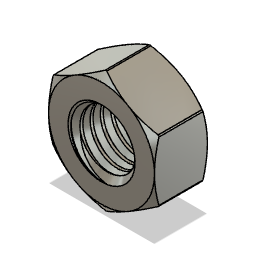
M8 Nut v5 (Autodesk Fusion 360 design; units mm, degrees)
Autodesk Fusion 360 part; units mm, degrees
sketch "Skizze1" plane through (0, 0, 0) normal (0, 0, 1) x (1, 0, 0)
  line L0 (-6.5, -3.7528) -> (0, -7.5056)
  line L1 (0, -7.5056) -> (6.5, -3.7528)
  line L2 (6.5, -3.7528) -> (6.5, 3.7528)
  line L3 (6.5, 3.7528) -> (0, 7.5056)
  line L4 (0, 7.5056) -> (-6.5, 3.7528)
  line L5 (-6.5, 3.7528) -> (-6.5, -3.7528)
  dimension "d3" = 6.5
  constraint vertical L5
  measures "d3" distance of origin L5
extrude "Extrusion1" add sketch "Skizze1" along normal mid plane 6.5
sketch "Skizze2" plane through (0, 0, 3.25) normal (0, 0, 1) x (1, 0, 0)
  line L0 (-6.5, 3.7528) -> (-6.5, -3.7528)
  line L1 (-6.5, -3.7528) -> (0, -7.5056)
  line L2 (0, -7.5056) -> (6.5, -3.7528)
  line L3 (6.5, -3.7528) -> (6.5, 3.7528)
  line L4 (6.5, 3.7528) -> (0, 7.5056)
  line L5 (0, 7.5056) -> (-6.5, 3.7528)
hole "Bohrung1" at (0, 0, 3.25) direction (0, 0, -1) diameter 6.78 end through all
thread "Gewinde1" "ISO Metric profile 8.0 M8x1.25 6H" major diameter 8.17 minor diameter 6.7795 pitch 1.25 angle 60 modelled right hand crest width 0.343 on face at (0.3375, -3.3732, -1.0833) crest through (3.3898, 0, 2.9375)
sketch "Skizze4" plane through (0, 0, 0) normal (1, 0, 0) x (0, 0, -1)
  line L0 (3.25, 3.7528) -> (3.25, 7.5056)
  line L1 (3.25, -3.7528) -> (3.25, 3.7528) construction
  line L2 (3.25, -7.5056) -> (3.25, -3.7528)
  line L3 (3.25, 7.5056) -> (-3.25, 7.5056)
  line L4 (2.6726, 7.5056) -> (3.25, 6.5056)
  line L5 (3.25, 7.5056) -> (2.817, 7.2556) construction
  line L6 (3.25, 6.5056) -> (3.25, 0)
  line L7 (2.6726, 7.5056) -> (0, 7.5056)
  line L8 (0, 1.75) -> (0, 22.5) construction
  line L9 (-2.6726, 7.5056) -> (0, 7.5056)
  line L10 (-2.6726, 7.5056) -> (-3.25, 6.5056)
  line L11 (-3.25, 6.5056) -> (-3.25, 0)
  line L12 (-3.25, 0) -> (3.25, 0)
  line L13 (-3.25, 8.5056) -> (0, 8.5056)
  line L14 (3.25, 8.5056) -> (0, 8.5056)
  line L15 (3.25, 8.5056) -> (4.25, 6.7735)
  line L16 (4.25, 6.7735) -> (4.25, -1)
  line L17 (-4.25, -1) -> (4.25, -1)
  line L18 (-4.25, 6.7735) -> (-4.25, -1)
  line L19 (-3.25, 8.5056) -> (-4.25, 6.7735)
  line L20 (-3.25, 0) -> (-4.25, 0)
  line L21 (3.25, 0) -> (4.25, 0)
  dimension "d18" = 0.5
  dimension "d19" = 1
  dimension "d23" = 150
  constraint coincident L3 L4.start
  constraint coincident L0 L4.end
  constraint coincident L0.end L3.start
  constraint midpoint L1 L6.end
  constraint midpoint L3 L7.end
  constraint symmetric L4.start L8 L9.start
  constraint symmetric L4.end L8 L10.end
  constraint symmetric L6.end L8 L11.end
  constraint symmetric L7.end L8 L9.end
  constraint coincident L18 L20.end
  constraint perpendicular L18 L20
  constraint coincident L16 L21.end
  constraint perpendicular L16 L21
  constraint perpendicular L4 L5
  constraint coincident L4 L5.end
  measures "d18" distance of L0.end L5.end
  measures "d23" angle of L4 L6
revolve "Drehen1" cut sketch "Skizze4" angle 360 about axis through (0, 0, 1.75) along (0, 0, 1) contours L0 L3 L6 L7 L9 L10 L11 L13 L14 L15 L16 L18 L19 L20 L21 | L0 L3 L4
fillet "Abrundung1" radius 0.2 6 edges at (6.5, 3.7528, 0) (6.5, -3.7528, 0) (0, -7.5056, 0) (-6.5, -3.7528, 0) (0, 7.5056, 0) (-6.5, 3.7528, 0)
sketch "Skizze5" plane through (0, 0, 0) normal (1, 0, 0) x (0, 0, -1)
  line L0 (-3.25, 4.1071) -> (-2.5429, 3.4)
  line L1 (-2.5429, 3.4) -> (0, 3.4)
  line L2 (0, 1.75) -> (0, 22.5)
  line L3 (0, 3.4) -> (0, 0) construction
  line L4 (-2.5429, 3.4) -> (-3.25, 3.4) construction
  line L5 (-3.25, 3.4) -> (-2.8964, 3.7536) construction
  line L6 (-3.25, 4.1071) -> (-3.25, 0)
  line L7 (-3.25, 0) -> (0, 0)
  line L8 (2.5429, 3.4) -> (0, 3.4)
  line L9 (3.25, 4.1071) -> (2.5429, 3.4)
  line L10 (3.25, 4.1071) -> (3.25, 0)
  line L11 (3.25, 0) -> (0, 0)
  line L12 (-3.25, -5.7635) -> (-3.25, -6.5056)
  line L13 (-3.25, -0.2687) -> (-3.25, -5.4948)
  line L14 (-3.25, 5.4948) -> (-3.25, 0.2687)
  line L15 (-3.25, 6.5056) -> (-3.25, 5.7635)
  line L16 (-3.25, 5.4948) -> (-3.25, 0.2687)
  line L17 (-3.25, -0.2687) -> (-3.25, -5.4948)
  dimension "d28" = 3.4
  dimension "d29" = 0.5
  dimension "d31" = 45
  constraint horizontal L1
  constraint coincident L1.end L2
  constraint coincident L3.end L7.end
  constraint coincident L0 L5.end
  constraint perpendicular L0 L5
  constraint symmetric L0.start L2 L9.start
  constraint symmetric L0.end L2 L8.start
  constraint symmetric L1.end L2 L3.start
  constraint symmetric L2 L6.end L10.end
  constraint symmetric L2 L3.end L7.end
  constraint horizontal L7
  constraint vertical L6
  constraint horizontal L4
  constraint coincident L4.end L6
  constraint collinear L6 L14
  measures "d28" distance of L1.end L3.end
  measures "d29" distance of L4.end L5.end
  measures "d31" angle of L0 L6
revolve "Drehen2" cut sketch "Skizze5" angle 360 about axis through (0, 0, 1.75) along (0, 0, 1)
equation "HexWidth = 13 mm" comment "Side-to-side width"
equation "Height = 6.5 mm"
equation "d3 = HexWidth / 2"
equation "d4 = Height"
equation "ChamferDepth = 0.5 mm" comment "Corner chamfer depth"
equation "ChamferAngle = 30 deg" comment "Corner chamfer angle"
equation "ThreadChamferDepth = 0.5 mm"
equation "d18 = ChamferDepth"
equation "d19 = 2 * ChamferDepth"
equation "SideFillet = 0.2 mm" comment "Fillet of the sides"
equation "d22 = SideFillet"
equation "d23 = 180 deg - ChamferAngle"
equation "ThreadChamferAngle = 45 deg"
equation "CoreDrill = 6.8 mm" comment "Core drill size for the given thread. Used to compute the thread chamfer."
equation "d28 = CoreDrill / 2"
equation "d29 = ThreadChamferDepth"
equation "d31 = ThreadChamferAngle"
named bodies: "Nut"
